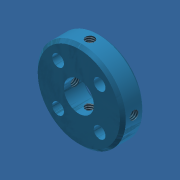
# Autodesk Inventor part: None_Magnet_Extender_Split_Bottom
Saved by Autodesk Inventor 2015 (Build 190159000, 159)
## iProperties
Created: 2015-01-06
Part Number: None_Magnet_Extender_Split_Bottom
Material: Aluminum 6061
Document SubType Name: Modeling
Designer: ice
Mass: 1.54881 g
Surface Area: 8.35285 cm^2
Volume: 0.573632 cm^3
Density: 2.7 g/cm^3
Appearance: Aluminum - Flat
Author: ice
Autodesk Inventor part; units mm, degrees
sketch "Sketch1" plane through (0, 0, 0) normal (1, 0, 0) x (0, 1, 0)
  line L0 (16.6, 2.55) -> (20.4, 2.55)
  line L1 (20.8521, 0) -> (14.3565, 0)
  line L2 (16.6, 7.5) -> (20.4, 7.5)
  line L3 (20.4, 7.5) -> (20.4, 2.55)
  line L4 (20.4, 5.025) -> (20.4, 2.55)
  line L5 (20.4, 7.5) -> (20.4, 7)
  line L6 (20.4, 7.5) -> (19.9, 7.5)
  line L7 (20.4, 2.55) -> (20.4, 3.05)
  line L8 (20.4, 2.55) -> (19.9, 2.55)
  line L9 (20.4, 7.5) -> (16.6, 7.5)
  line L10 (16.6, 7.5) -> (16.6, 2.55)
  point P0 (0, 0)
  dimension "d267" = 5.025
  dimension "d306" = 7.5
  dimension "d339" = 0.5
  dimension "d340" = 0.5
  dimension "d341" = 0.5
  dimension "d342" = 0.5
  dimension "d350" = 3.8
  constraints: 22 end point, 4 point on line, 2 perpendicular, 1 collinear, 1 horizontal, 1 midpoint
  measures "d267" distance from line of L1 L4.start
  measures "d306" vertical distance of L1.start L2.end
  measures "d339" distance of L2.end L5.end
  measures "d340" distance of L2.end L6.end
  measures "d341" distance of L0.end L7.end
  measures "d342" distance of L0.end L8.end
  measures "d350" distance of L2.start L2.end
revolve "Revolution1" add sketch "Sketch1" angle 360 about axis through (0, 20.8521, 0) along (0, -1, 0)
ref_plane "Work Plane12" through (0, 0, 5) normal (0, 0, 1) x (1, 0, 0)
ref_plane "Work Plane3" through (5, 0, 0) normal (1, 0, 0) x (0, 1, 0)
sketch "Sketch10" plane through (0, 20.4, 0) normal (0, 1, 0) x (1, 0, 0)
  line L0 (0, 0) -> (2.55, 0)
  circle A0 centre (0, 0) radius 2.55 projected
  line L1 (2.55, 0) -> (7.5, 0)
  circle A1 centre (0, 0) radius 7.5 projected
  line L2 (0, 0) -> (3.5355, -3.5355)
  line L3 (0, 0) -> (5, 0) construction
  line L4 (0, 0) -> (3.5355, 3.5355)
  line L5 (0, 0) -> (-3.5355, 3.5355)
  line L6 (0, 0) -> (5, 0) construction
  line L7 (0, 0) -> (-3.5355, -3.5355)
  line L8 (0, 0) -> (5, 0) construction
  circle A2 centre (3.5355, 3.5355) radius 1
  circle A3 centre (-3.5355, 3.5355) radius 1
  circle A4 centre (-3.5355, -3.5355) radius 1
  circle A5 centre (3.5355, -3.5355) radius 1
  line L9 (0, 0) -> (0, -5)
  line L10 (0, 0) -> (-5, 0)
  line L11 (0, 0) -> (0, 5)
  dimension "d268" = 4.95
  dimension "d269" = 2.55
  dimension "d270" = 5
  dimension "d271" = 45
  dimension "d272" = 5
  dimension "d273" = 5
  dimension "d275" = 5
  dimension "d335" = 2
  dimension "d336" = 2
  dimension "d337" = 2
  dimension "d338" = 2
  dimension "d376" = 5
  dimension "d377" = 5
  dimension "d378" = 5
  dimension "d379" = 45
  dimension "d380" = 45
  dimension "d381" = 90
  dimension "d382" = 45
  dimension "d383" = 45
  dimension "d384" = 45
  dimension "d385" = 45
  dimension "d386" = 45
  dimension "d387" = 90
  constraints: 24 end point, 4 centre point, 4 horizontal, 3 coincident, 3 equal length, 2 horizontal alignment, 2 point on line, 2 vertical, 1 perpendicular, 2 other
  measures "d268" distance of L0.end L1.end
  measures "d269" distance of L0.end L0.start
  measures "d270" distance of L2.start L2.end
  measures "d271" angle of L2 L3
  measures "d272" distance of L2.start L4.end
  measures "d273" distance of L2.start L5.end
  measures "d275" distance of L2.start L7.end
  measures "d335" diameter of A2
  measures "d336" diameter of A3
  measures "d337" diameter of A4
  measures "d338" diameter of A5
  measures "d376" distance of L2.start L9.end
  measures "d377" distance of L2.start L10.end
  measures "d378" distance of L2.start L11.end
  measures "d379" angle of L4 L3
  measures "d380" angle of L11 L4
  measures "d381" angle of L11 L3
  measures "d382" angle of L11 L5
  measures "d383" angle of L10 L5
  measures "d384" angle of L7 L10
  measures "d385" angle of L7 L9
  measures "d386" angle of L2 L9
  measures "d387" angle of L10 L9
hole "Hole6" at (3.5355, 20.4, -3.5355) at (3.5355, 20.4, 3.5355) at (-3.5355, 20.4, 3.5355) at (-3.5355, 20.4, -3.5355) direction (0, -1, 0) diameter 2 end through all counterbore diameter 4.1 counterbore depth 1.8
ref_plane "Work Plane15" through (0, 0, 7.5) normal (0, 0, 1) x (1, 0, 0)
sketch "Sketch12" plane through (0, 0, 7.5) normal (0, 0, 1) x (1, 0, 0)
  line L0 (-2.55, 16.6) -> (2.55, 16.6) projected
  line L1 (-7.5, 20.4) -> (7.5, 20.4) projected
  line L2 (0, 18.5) -> (0, 16.6)
  point P0 (0, 17.65)
  constraints: 2 end point, 1 midpoint
ref_plane "Work Plane8" through (7.5, 0, 0) normal (1, 0, 0) x (0, 1, 0)
sketch "Sketch13" plane through (7.5, 0, 0) normal (1, 0, 0) x (0, 1, 0)
  line L0 (20.4, 7.5) -> (20.4, -7.5) projected
  line L1 (15.4, 7.5) -> (15.4, -7.5) projected
  line L2 (15.4, 0) -> (17.65, 0)
  line L3 (20.4, 0) -> (16.6, 0)
  line L4 (16.6, 0) -> (18.5, 0)
  point P0 (0, 0)
  dimension "d352" = 1.9
  constraints: 6 end point, 3 midpoint
  measures "d352" distance of L3.end L4.end
chamfer "Chamfer5" distance 0.5 angle 45 3 edges at (0, 20.4, -7.5) (0, 20.4, -2.55) (0, 16.6, -7.5)
ref_plane "Work Plane16" through (-3.5355, 18.6, -3.5355) normal (0, 1, 0) x (1, 0, 0)
ref_plane "Work Plane17" through (3.5355, 18.6, -3.5355) normal (0, 1, 0) x (1, 0, 0)
ref_plane "Work Plane18" through (-3.5355, 18.6, 3.5355) normal (0, 1, 0) x (1, 0, 0)
ref_plane "Work Plane19" through (3.5355, 18.6, 3.5355) normal (0, 1, 0) x (1, 0, 0)
hole "Hole9" at (7.5, 18.5, 0) direction (-1, 0, 0) diameter 1.5 end through all
hole "Hole10" at (0, 18.5, 7.5) direction (0, 0, -1) diameter 1.5 end through all
thread "Thread19" size "M1.6x0.35" class "6H" standard "ANSI Metric M Profile" full length
thread "Thread20" size "M1.6x0.35" class "6H" standard "ANSI Metric M Profile" full length
thread "Thread21" size "M1.6x0.35" class "6H" standard "ANSI Metric M Profile" full length
thread "Thread22" size "M1.6x0.35" class "6H" standard "ANSI Metric M Profile" full length
ref_plane "Work Plane25" through (0, 16.6, 0) normal (0, -1, 0) x (1, 0, 0)
ref_plane "Work Plane21" through (0, 0, -2.5) normal (0, 0, 1) x (1, 0, 0)
ref_plane "Work Plane20" through (0, 0, 2.5) normal (0, 0, 1) x (1, 0, 0)
ref_plane "Work Plane23" through (-2.5, 0, 0) normal (1, 0, 0) x (0, 1, 0)
ref_plane "Work Plane22" through (2.5, 0, 0) normal (1, 0, 0) x (0, 1, 0)
body "Solid1"
